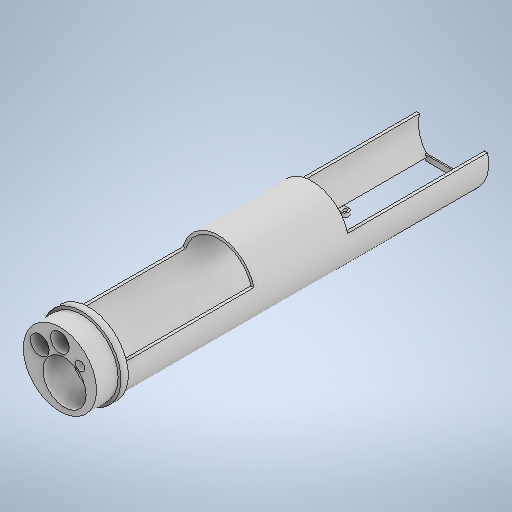
# Autodesk Inventor part: PCB tray CAD
Saved by Autodesk Inventor 2025 (Build 290162000, 162)
## iProperties
Created: 2024-07-01
Part Number: PCB tray CAD
Material: Generic
Document SubType Name: Modeling
Designer: track
Density: 1 g/cm^3
Appearance: Default
Author: track
## iProperties of the stored document PCB tray CAD_3DPrint.ipt
Created: 2024-07-01
Part Number: PCB tray CAD_3DPrint
Material: Generic
Document SubType Name: Modeling
Designer: track
Density: 1 g/cm^3
Appearance: Default
Author: track
Autodesk Inventor part; units mm, degrees
ref_plane "YZ Plane" through (0, 0, 0) normal (1, 0, 0) x (0, 1, 0)
ref_plane "XY Plane" through (0, 0, 0) normal (0, 0, 1) x (1, 0, 0)
sketch "Sketch9" plane through (0, 0, 0) normal (0, 0, 1) x (1, 0, 0)
  circle A0 centre (0, 0) radius 25.4
  circle A1 centre (0, 0) radius 23.4
  dimension "d29" = 50.8
  dimension "d30" = 2
  constraints: 2 centre point, 2 coincident
  measures "d29" diameter of A0
  measures "d30" radial gap between concentric circles of A0 A1
extrude "Extrusion7" add sketch "Sketch9" against normal blind 272
sketch "Sketch10" plane through (0, 0, 0) normal (0, 0, 1) x (1, 0, 0)
  circle A0 centre (0, 16.129) radius 6.5
  circle A1 centre (-13.97, 7.62) radius 6.5
  circle A2 centre (13.97, 8.89) radius 3.25
  circle A3 centre (0, 0) radius 23.4 projected
  circle A4 centre (3.175, -6.35) radius 15
  dimension "d33" = 13
  dimension "d34" = 13
  dimension "d35" = 6.5
  dimension "d77" = 30
  dimension "d78" = 3.175
  dimension "d79" = 6.35
  dimension "d80" = 8.89
  dimension "d81" = 13.97
  dimension "d82" = 0
  dimension "d83" = 16.129
  dimension "d84" = 13.97
  dimension "d85" = 7.62
  constraints: 4 centre point
  measures "d33" diameter of A0
  measures "d34" diameter of A1
  measures "d35" diameter of A2
  measures "d77" diameter of A4
  measures "d78" horizontal distance of A4.centre point (0, 0)
  measures "d79" vertical distance of point (0, 0) A4.centre
  measures "d80" vertical distance of A2.centre point (0, 0)
  measures "d81" horizontal distance of point (0, 0) A2.centre
  measures "d82" horizontal distance of point (0, 0) A0.centre
  measures "d83" distance of point (0, 0) A0.centre
  measures "d84" horizontal distance of point (0, 0) A1.centre
  measures "d85" vertical distance of point (0, 0) A1.centre
extrude "Extrusion8" add sketch "Sketch10" against normal blind 20
ref_plane "Work Plane1" through (0, 25.4, 0) normal (0, 1, 0) x (-1, 0, 0)
sketch "Sketch11" plane through (0, 25.4, 0) normal (0, 1, 0) x (-1, 0, 0)
  line L0 (-25.4, -272) -> (25.4, -272) projected
  line L1 (-25.4, 0) -> (-25.4, -272) projected
  line L2 (25.4, -272) -> (-25.4, -272)
  line L3 (-25.4, -272) -> (-25.4, -175)
  line L4 (-25.4, -175) -> (25.4, -175)
  line L5 (25.4, -175) -> (25.4, -272)
  point P0 (0, 0)
  dimension "d53" = 97
  constraints: 8 end point, 2 parallel, 1 horizontal, 1 perpendicular, 1 point on line
  measures "d53" distance of L4.end L0.end
extrude "Extrusion9" cut sketch "Sketch11" against normal blind 19.05
sketch "Sketch12" plane through (0, 0, -272) normal (0, 0, -1) x (-1, 0, 0)
  circle A0 centre (0, 0) radius 25.4 projected
  line L0 (-19.2809, -16.535) -> (19.2809, -16.535)
  line L1 (16, -16.535) -> (-16, -16.535) projected
  arc A1 (-19.2809, -16.535) -> (19.2809, -16.535) centre (0, 0) ccw
  dimension "d86" = 16.535
  constraints: 4 point on circle, 2 end point, 1 centre point, 1 concentric, 1 horizontal
  measures "d86" distance from line of A0.centre L0
extrude "Extrusion10" cut sketch "Sketch12" against normal blind 97 contours L0 A0 picked at (1.0399, -19.4259)
ref_plane "Work Plane3" through (0, -16.51, 0) normal (0, 1, 0) x (-1, 0, 0)
sketch "Sketch13" plane through (0, -16.51, 0) normal (0, 1, 0) x (-1, 0, 0)
  line L0 (0, 0) -> (0, -257.1233) construction
  line L1 (-16.5576, -272) -> (-16.5576, -175) projected
  line L2 (-16.5576, -175) -> (-13.0576, -175)
  line L3 (-13.0576, -175) -> (-13.0576, -180) construction
  line L4 (-13.0576, -180) -> (-16.5576, -180)
  line L5 (-16.5576, -180) -> (-16.5576, -175)
  line L6 (16.5576, -175) -> (16.5576, -272) projected
  line L7 (16.5576, -175) -> (13.0576, -175)
  line L8 (13.0576, -175) -> (13.0576, -180) construction
  line L9 (13.0576, -180) -> (16.5576, -180)
  line L10 (16.5576, -180) -> (16.5576, -175)
  line L11 (-16.5576, -208.5) -> (-13.0576, -208.5)
  line L12 (-13.0576, -208.5) -> (-13.0576, -213.5) construction
  line L13 (-13.0576, -213.5) -> (-16.5576, -213.5)
  line L14 (-16.5576, -213.5) -> (-16.5576, -208.5)
  line L15 (16.5576, -208.5) -> (13.0576, -208.5)
  line L16 (13.0576, -208.5) -> (13.0576, -213.5) construction
  line L17 (13.0576, -213.5) -> (16.5576, -213.5)
  line L18 (16.5576, -213.5) -> (16.5576, -208.5)
  arc A0 (-13.0576, -180) -> (-13.0576, -175) centre (-13.0576, -177.5) ccw
  arc A1 (13.0576, -175) -> (13.0576, -180) centre (13.0576, -177.5) ccw
  arc A2 (-13.0576, -213.5) -> (-13.0576, -208.5) centre (-13.0576, -211) ccw
  arc A3 (13.0576, -208.5) -> (13.0576, -213.5) centre (13.0576, -211) ccw
  circle A4 centre (-13.0576, -177.5) radius 1.25
  circle A5 centre (13.0576, -177.5) radius 1.25
  circle A6 centre (-13.0576, -211) radius 1.25
  circle A7 centre (13.0576, -211) radius 1.25
  point P0 (-10.5576, -177.5)
  point P1 (16.5576, -213.5)
  point P2 (16.5576, -208.5)
  point P3 (-16.5576, -208.5)
  point P4 (-16.5576, -213.5)
  dimension "d60" = 5
  dimension "d61" = 5
  dimension "d62" = 28.5
  dimension "d63" = 6
  dimension "d64" = 2.5
  dimension "d65" = 2.5
  constraints: 34 end point, 9 point on circle, 8 centre point, 8 parallel, 8 tangent, 5 point on line, 4 coincident, 4 horizontal, 4 perpendicular, 1 vertical, 6 other
  measures "d60" distance of L2.end L3.end
  measures "d61" distance of L11.end L12.end
  measures "d62" distance between parallel lines of L4 L11
  measures "d63" distance from line of L1 point (-10.558, -177.5)
  measures "d64" diameter of A4
  measures "d65" diameter of A6
extrude "Extrusion11" add sketch "Sketch13" against normal blind 2.54
sketch "Sketch14" plane through (0, 0, -175) normal (0, 0, -1) x (-1, 0, 0)
  line L0 (16.5576, -19.05) -> (13.5889, -19.05) projected
  arc A0 (-13.5889, -19.05) -> (13.5889, -19.05) centre (0, 0) ccw projected
  line L1 (-13.5889, -19.05) -> (-16.5576, -19.05) projected
  line L2 (-16.5576, -19.05) -> (-16.5576, -16.535) projected
  line L3 (-19.2809, -16.535) -> (-16.5576, -16.535) projected
  arc A1 (-19.2809, -16.535) -> (19.2809, -16.535) centre (0, 0) ccw projected
  line L4 (16.5576, -16.535) -> (19.2809, -16.535) projected
  line L5 (16.5576, -16.535) -> (16.5576, -19.05) projected
  line L6 (13.0576, -16.51) -> (13.0576, -19.05) projected
  line L7 (13.0576, -19.05) -> (16.8005, -19.05)
  line L8 (-13.0576, -16.51) -> (-13.0576, -19.05) projected
  line L9 (-13.0576, -19.05) -> (-16.8005, -19.05)
  point P0 (-16.5576, -19.2615)
  point P1 (16.5576, -19.2615)
  constraints: 4 end point, 4 point on circle, 3 point on line, 1 perpendicular
extrude "Extrusion12" add sketch "Sketch14" along normal up to surface (38.5 mm away) contours L5 L4 A1 L7 | A1 L3 L2 L9
sketch "Sketch15" plane through (0, 25.4, 0) normal (0, 1, 0) x (-1, 0, 0)
  line L0 (-25.4, 0) -> (-25.4, -272) projected
  line L1 (25.4, 0) -> (25.4, -272) projected
  line L2 (-25.4, -20) -> (25.4, -20)
  line L3 (25.4, -20) -> (25.4, -110)
  line L4 (25.4, -110) -> (-25.4, -110)
  line L5 (-25.4, -110) -> (-25.4, -20)
  line L6 (23.4, -20) -> (-23.4, -20) projected
  point P0 (0, 0)
  point P1 (-25.4, -110)
  point P2 (25.4, -20)
  dimension "d70" = 0
  dimension "d71" = 90
  constraints: 8 end point, 2 parallel, 2 point on line, 1 horizontal, 1 perpendicular
  measures "d70" distance between parallel lines of L6 L2
  measures "d71" distance between parallel lines of L2 L4
extrude "Extrusion13" cut sketch "Sketch15" against normal up to surface (19.05 mm away)
sketch "Sketch17" plane through (0, 0, -272) normal (0, 0, -1) x (-1, 0, 0)
  circle A0 centre (0, 0) radius 25.4
  arc A1 (-16.8005, -19.05) -> (16.8005, -19.05) centre (0, 0) ccw projected
  line L0 (-19.2809, -16.535) -> (-16.5576, -16.535) projected
  line L1 (-20.32, -15.24) -> (20.32, -15.24)
  line L2 (16.5576, -19.05) -> (13.0576, -19.05) projected
  line L3 (-16.8005, -19.05) -> (16.8005, -19.05)
  point P0 (16.8005, -19.05)
  dimension "d74" = 3.81
  constraints: 4 end point, 2 parallel, 2 point on circle, 1 centre point, 1 coincident, 1 concentric
  measures "d74" distance between parallel lines of L1 L3
extrude "Extrusion14" add sketch "Sketch17" against normal blind 1 contours L1 A0 L3 L2
sketch "Sketch18" plane through (0, 0, -20) normal (0, 0, -1) x (-1, 0, 0)
  circle A0 centre (0, 0) radius 27.4
  circle A1 centre (0, 0) radius 25.4
  arc A2 (16.8005, -19.05) -> (24.5934, 6.35) centre (0, 0) ccw projected
  dimension "d87" = 2
  constraints: 2 centre point, 2 coincident, 1 concentric
  measures "d87" radial gap between concentric circles of A0 A1
extrude "Extrusion15" add sketch "Sketch18" against normal blind 5
body "Solid2"
